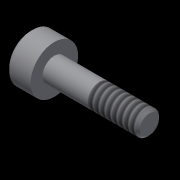
# Autodesk Inventor part: Bolt1
Saved by Autodesk Inventor 2020 (Build 240168000, 168)
## iProperties
Created: 2010-08-06
Part Number: Bolt1
Document SubType Name: Modeling
Designer: nguyenducthang
Density: 1 g/cm^3
Mass: 0.00563194 g
Surface Area: 0.269795 cm^2
Volume: 0.00563194 cm^3
Material: 一般
Appearance: 預設
Author: nguyenducthang
Autodesk Inventor part; units mm, degrees
ref_plane "YZ Plane" through (0, 0, 0) normal (1, 0, 0) x (0, 1, 0)
ref_plane "XZ Plane" through (0, 0, 0) normal (0, 1, 0) x (-1, 0, 0)
ref_plane "XY Plane" through (0, 0, 0) normal (0, 0, 1) x (1, 0, 0)
sketch "Sketch15" plane through (0, 0, 0) normal (0, 0, 1) x (1, 0, 0)
  line L0 (0, 0) -> (0, 1)
  line L1 (0, 1) -> (1, 1)
  line L2 (3, 4.4) -> (3, 4.4)
  line L3 (1, 0.5) -> (5, 0.5)
  line L4 (5, 0) -> (0, 0)
  line L5 (1, 0.5) -> (1, 1)
  line L6 (5, 0.5) -> (5, 0)
  dimension "d84" = 0.5
  dimension "d87" = 1
  dimension "d116" = 1
  dimension "d117" = 4
  constraints: 14 end point, 4 parallel, 1 perpendicular, 1 vertical, 1 other
  measures "d84" distance between parallel lines of L3 L4
  measures "d87" distance between parallel lines of L1 L4
  measures "d116" distance between parallel lines of L0 L5
  measures "d117" distance of L3.start L3.end
revolve "Revolution1" add sketch "Sketch15" angle 360 about axis through (5, 0, 0) along (-1, 0, 0)
chamfer "Chamfer5" distance 0.1 angle 45 1 edges at (5, -0.5, 0)
thread "Thread8" size "M1x0.25" class "6g" standard "ANSI Metric M Profile" length 2
chamfer "Chamfer6" distance 0.1 angle 45 1 edges at (0, -1, 0)
sketch "Sketch19" plane through (0, 0, 0) normal (-1, 0, 0) x (0, 0, 1)
  circle A0 centre (0, 0) radius 0.9 projected
  line L0 (0.2887, 0.5) -> (0.5774, 0)
  line L1 (0.5774, 0) -> (0.2887, -0.5)
  line L2 (0.2887, -0.5) -> (-0.2887, -0.5)
  line L3 (-0.2887, -0.5) -> (-0.5774, 0)
  line L4 (-0.5774, 0) -> (-0.2887, 0.5)
  line L5 (-0.2887, 0.5) -> (0.2887, 0.5)
  dimension "d137" = 1
  constraints: 12 end point, 1 coincident, 13 other
  measures "d137" distance between parallel lines of L2 L5
extrude "Extrusion18" cut sketch "Sketch19" against normal blind 0.7 contours L0 L1 L2 L3 L4 L5
